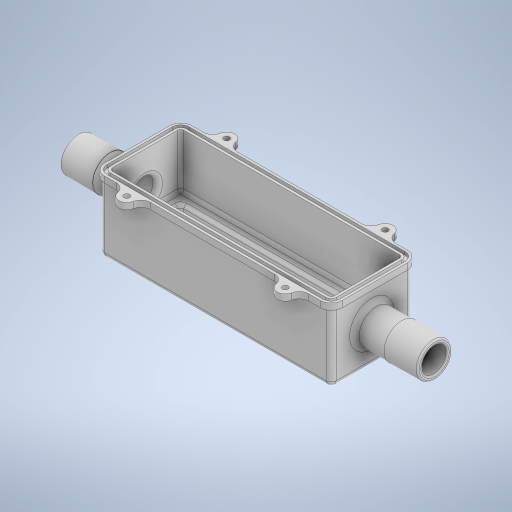
# Autodesk Inventor part: Rebreather-SensorEnclosure-v2
Saved by Autodesk Inventor 2023 (Build 270158000, 158)
## iProperties
Created: 2022-11-09
Part Number: Rebreather-SensorEnclosure-v2
Material: Generic
Document SubType Name: Modeling
Designer: incep
Density: 1 g/cm^3
Appearance: Default
Author: incep
## iProperties of the stored document Rebreather-SensorEnclosure_3DPrint.ipt
Created: 2022-11-09
Part Number: Rebreather-SensorEnclosure_3DPrint
Material: Generic
Document SubType Name: Modeling
Designer: incep
Density: 1 g/cm^3
Appearance: Default
Author: incep
Autodesk Inventor part; units mm, degrees
ref_plane "YZ Plane" through (0, 0, 0) normal (1, 0, 0) x (0, 1, 0)
ref_plane "XZ Plane" through (0, 0, 0) normal (0, 1, 0) x (-1, 0, 0)
sketch "Sketch1" plane through (0, 0, 0) normal (0, 1, 0) x (-1, 0, 0)
  line L0 (62.5, -15) -> (-62.5, -15) construction
  line L1 (-62.5, -15) -> (-62.5, 15) construction
  line L2 (-62.5, 15) -> (62.5, 15) construction
  line L3 (62.5, 15) -> (62.5, -15) construction
  line L4 (63, -15.5) -> (-63, -15.5)
  line L5 (-63, -15.5) -> (-63, 15.5)
  line L6 (-63, 15.5) -> (63, 15.5)
  line L7 (63, 15.5) -> (63, -15.5)
  line L8 (73, -25.5) -> (-73, -25.5)
  line L9 (-73, -25.5) -> (-73, 25.5)
  line L10 (-73, 25.5) -> (73, 25.5)
  line L11 (73, 25.5) -> (73, -25.5)
  line L12 (70, -22.5) -> (-70, -22.5)
  line L13 (-70, -22.5) -> (-70, 22.5)
  line L14 (-70, 22.5) -> (70, 22.5)
  line L15 (70, 22.5) -> (70, -22.5)
  point P0 (0, 0)
  point P1 (-62.5, 0)
  point P2 (0, -15)
  point P3 (-63, 0)
  point P4 (0, -15.5)
  point P5 (0, -25.5)
  point P6 (-73, 0)
  point P7 (0, -22.5)
  point P8 (-70, 0)
  dimension "d0" = 125
  dimension "d1" = 30
  dimension "d2" = 0.5
  dimension "d3" = 0.5
  dimension "d4" = 10
  dimension "d5" = 10
  dimension "d6" = 3
  dimension "d7" = 3
  constraints: 32 end point, 8 midpoint, 8 parallel, 4 horizontal, 4 horizontal alignment, 4 perpendicular, 4 vertical alignment
  measures "d0" distance of L1.end L2.end
  measures "d1" distance of L0.end L1.end
  measures "d2" distance between parallel lines of L7 L3
  measures "d3" distance between parallel lines of L4 L0
  measures "d4" distance between parallel lines of L11 L7
  measures "d5" distance between parallel lines of L8 L4
  measures "d6" distance between parallel lines of L15 L11
  measures "d7" distance between parallel lines of L8 L12
extrude "Extrusion1" add sketch "Sketch1" along normal blind 40 contours L8 L9 L10 L11
extrude "Extrusion2" add sketch "Sketch1" along normal blind 10 contours L12 L13 L14 L15
extrude "Extrusion3" add sketch "Sketch1" against normal blind 3 contours L4 L5 L6 L7 | L8 L9 L10 L11 | L12 L13 L14 L15
sketch "Sketch2" plane through (73, 40, 25.5) normal (1, 0, 0) x (0, 0, -1)
  line L0 (0, -43) -> (0, 0) projected
  line L1 (0, 0) -> (51, 0) projected
  line L2 (51, -43) -> (51, 0) projected
  line L3 (51, -40) -> (0, -40) projected
  line L4 (51, 0) -> (0, 0) construction
  line L5 (25.5, 0) -> (25.5, -40) construction
  line L6 (41, -40) -> (10, -40) construction
  line L7 (0, 0) -> (0, -43) construction
  line L8 (0, -20) -> (51, -20) construction
  line L9 (51, -43) -> (51, 0) construction
  point P0 (25.5, -20)
  point P1 (25.5, -20)
  constraints: 4 end point, 3 midpoint, 2 perpendicular, 2 point on line, 1 coincident
ref_plane "Work Plane1" through (-73, 40, 0) normal (0, 0, 1) x (1, 0, 0)
sketch "Sketch3" plane through (-73, 40, 0) normal (0, 0, 1) x (1, 0, 0)
  line L0 (186, -9.08) -> (146, -9.08) construction
  line L1 (146, -9.08) -> (146, -12.08)
  line L2 (146, -12.08) -> (186, -12.08)
  line L3 (186, -12.08) -> (186, -9.08)
  line L4 (146, -43) -> (146, 0) projected
  line L5 (186, -9.08) -> (165, -8.81)
  line L6 (165, -8.81) -> (165, -9.08)
  line L7 (165, -9.08) -> (146, -9.08)
  line L8 (146, -20) -> (225.0991, -20) construction
  point P0 (73, -40)
  dimension "d14" = 3
  dimension "d15" = 40
  dimension "d16" = 10.92
  dimension "d17" = 21
  dimension "d18" = 11.19
  constraints: 16 end point, 3 perpendicular, 2 horizontal, 2 parallel, 1 collinear, 1 point on line
  measures "d14" distance between parallel lines of L2 L0
  measures "d15" distance of L0.start L0.end
  measures "d16" vertical distance of L0.start L8.start
  measures "d17" horizontal distance of L5.end L0.start
  measures "d18" vertical distance of L8.start L5.end
revolve "Revolution1" add sketch "Sketch3" angle 360 about axis through (73, 20, 0) along (1, 0, 0)
sketch "Sketch4" plane through (73, 20, 0) normal (1, 0, 0) x (0, 0, -1)
  circle A0 centre (0, 0) radius 7.92 projected
  point P0 (0, -20)
extrude "Extrusion4" cut sketch "Sketch4" against normal up to surface (146 mm away)
mirror "Mirror1" about plane through (0, 0, 0) normal (1, 0, 0) of "Revolution1"
sketch "Sketch5" plane through (0, 40, 0) normal (0, 1, 0) x (1, 0, 0)
  line L0 (-75, 27.5) -> (75, 27.5)
  line L1 (75, 27.5) -> (75, -27.5)
  line L2 (75, -27.5) -> (-75, -27.5)
  line L3 (-75, -27.5) -> (-75, 27.5)
  line L4 (-70, 22.5) -> (70, 22.5) projected
  line L5 (-70, -22.5) -> (-70, 22.5) projected
  line L6 (70, -22.5) -> (-70, -22.5) projected
  line L7 (70, 22.5) -> (70, -22.5) projected
  point P0 (0, 0)
  point P1 (75, 0)
  point P2 (0, 27.5)
  dimension "d22" = 5
  dimension "d23" = 5
  constraints: 8 end point, 2 midpoint, 2 parallel, 1 horizontal, 1 horizontal alignment, 1 perpendicular, 1 vertical alignment
  measures "d22" distance between parallel lines of L0 L4
  measures "d23" distance between parallel lines of L3 L5
extrude "Extrusion5" add sketch "Sketch5" along normal blind 4
sketch "Sketch6" plane through (0, 44, 0) normal (0, 1, 0) x (1, 0, 0)
  line L0 (-75, 27.5) -> (-75, -27.5) projected
  line L1 (75, 27.5) -> (-75, 27.5) projected
  line L2 (75, -27.5) -> (75, 27.5) projected
  line L3 (-75, -27.5) -> (75, -27.5) projected
  line L4 (-73.5, 26) -> (73.5, 26)
  line L5 (73.5, 26) -> (73.5, -26)
  line L6 (73.5, -26) -> (-73.5, -26)
  line L7 (-73.5, -26) -> (-73.5, 26)
  line L8 (-71.5, 24) -> (71.5, 24)
  line L9 (71.5, 24) -> (71.5, -24)
  line L10 (71.5, -24) -> (-71.5, -24)
  line L11 (-71.5, -24) -> (-71.5, 24)
  point P0 (0, 0)
  point P1 (73.5, 0)
  point P2 (0, 26)
  point P3 (71.5, 0)
  point P4 (0, 24)
  dimension "d26" = 1.5
  dimension "d27" = 1.5
  dimension "d28" = 2
  dimension "d29" = 2
  constraints: 16 end point, 4 midpoint, 4 parallel, 2 horizontal, 2 horizontal alignment, 2 perpendicular, 2 vertical alignment
  measures "d26" distance between parallel lines of L0 L7
  measures "d27" distance between parallel lines of L1 L4
  measures "d28" distance between parallel lines of L4 L8
  measures "d29" distance between parallel lines of L7 L11
extrude "Extrusion6" cut sketch "Sketch6" against normal blind 2 contours L4 L5 L6 L7
sketch "Sketch7" plane through (0, 44, 0) normal (0, 1, 0) x (1, 0, 0)
  line L0 (-50, 31.5) -> (50, 31.5) construction
  line L1 (50, 31.5) -> (50, -31.5) construction
  line L2 (50, -31.5) -> (-50, -31.5) construction
  line L3 (-50, -31.5) -> (-50, 31.5) construction
  line L4 (-73, -25.5) -> (73, -25.5) construction
  circle A0 centre (-50, -31.5) radius 1.8
  circle A1 centre (-50, -31.5) radius 4.9833 construction
  line L5 (-75, -27.5) -> (75, -27.5) projected
  line L6 (-52.9721, -27.5) -> (-47.0279, -27.5)
  arc A2 (-52.9721, -27.5) -> (-47.0279, -27.5) centre (-50, -31.5) ccw
  point P0 (0, 0)
  point P1 (50, 0)
  point P2 (0, 31.5)
  dimension "d32" = 100
  dimension "d33" = 6
  dimension "d34" = 3.6
  dimension "d37" = 31.5
  constraints: 10 end point, 4 point on circle, 3 centre point, 3 coincident, 2 midpoint, 2 parallel, 2 point on line, 1 concentric, 1 horizontal, 1 horizontal alignment, 1 perpendicular, 1 vertical alignment
  measures "d32" distance of L1.end L2.end
  measures "d33" distance between parallel lines of L2 L4
  measures "d34" diameter of A0
  measures "d37" vertical distance of L2.end point (0, 0)
extrude "Extrusion7" add sketch "Sketch7" against normal up to surface (4 mm away)
mirror "Mirror2" about plane through (0, 0, 0) normal (1, 0, 0) of "Extrusion7"
mirror "Mirror3" about plane through (0, 0, 0) normal (0, 0, 1) of "Extrusion7", "Mirror2"
fillet "Fillet1" radius 6 8 edges at (-52.9721, 42, -27.5) (-47.0279, 42, -27.5) (52.9721, 42, -27.5) (47.0279, 42, -27.5) (52.9721, 42, 27.5) (47.0279, 42, 27.5) (-47.0279, 42, 27.5) (-52.9721, 42, 27.5)
fillet "Fillet2" radius 3 10 edges at (-73, 18.5, 25.5) (-73, -3, 0) (-73, 18.5, -25.5) (0, -3, 25.5) (-73, 9.08, 0) (73, 18.5, 25.5) (73, -3, 0) (73, 18.5, -25.5) (73, 9.08, 0) (0, -3, -25.5)
fillet "Fillet3" radius 1 4 edges at (113, 9.08, 0) (-113, 9.08, 0) (-113, 12.08, 0) (113, 12.08, 0)
fillet "Fillet4" radius 2 16 edges at (70, 27, 22.5) (70, 27, -22.5) (-70, 27, 22.5) (-70, 27, -22.5) (0, 10, -22.5) (0, 10, 22.5) (-70, 10, 0) (70, 10, 0) (63, 5, -15.5) (63, 5, 15.5) (-63, 5, -15.5) (-63, 5, 15.5) (0, 10, -15.5) (63, 10, 0) (0, 10, 15.5) (-63, 10, 0)
fillet "Fillet5" radius 3.5 4 edges at (71.5, 43, 24) (71.5, 43, -24) (-71.5, 43, -24) (-71.5, 43, 24)
fillet "Fillet6" radius 5.5 4 edges at (73.5, 43, 26) (73.5, 43, -26) (-73.5, 43, 26) (-73.5, 43, -26)
fillet "Fillet7" radius 7 4 edges at (-75, 42, -27.5) (-75, 42, 27.5) (75, 42, -27.5) (75, 42, 27.5)
fillet "Fillet8" radius 3 2 edges at (70, 20, 7.92) (-70, 20, 7.92)
body "Solid1"
